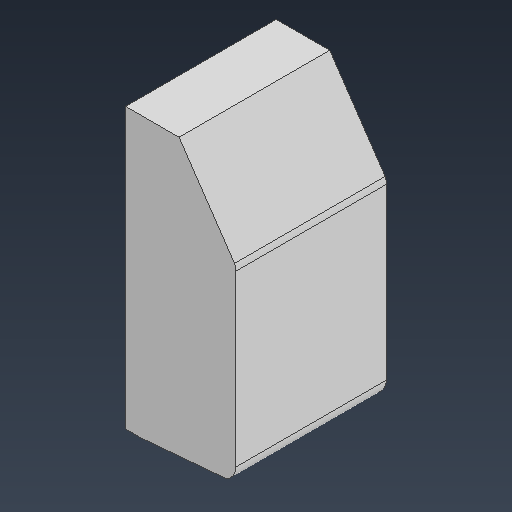
# Autodesk Inventor part: говно деда
Saved by Autodesk Inventor 2025 (Build 290162000, 162)
## iProperties
Created: 2025-03-14
Part Number: говно деда
Material: Типовые
Document SubType Name: Modeling
Designer: GameHD
Density: 1 g/cm^3
Appearance: По умолчанию
Author: GameHD
Autodesk Inventor part; units mm, degrees
ref_plane "YZ Plane" through (0, 0, 0) normal (1, 0, 0) x (0, 1, 0)
ref_plane "XZ Plane" through (0, 0, 0) normal (0, 1, 0) x (-1, 0, 0)
ref_plane "XY Plane" through (0, 0, 0) normal (0, 0, 1) x (1, 0, 0)
sketch "Эскиз1" plane through (0, 0, 0) normal (0, 0, 1) x (1, 0, 0)
  line L0 (-34.5939, -55.1342) -> (-34.5939, -82.0742)
  line L1 (-34.5939, -82.0742) -> (-25.3439, -82.0742)
  line L2 (-25.3439, -82.0742) -> (27.5337, -77.5454)
  arc A0 (27.5337, -77.5454) -> (33.4061, -68.437) centre (23.4061, -68.437) ccw
  line L3 (33.4061, -68.437) -> (33.4061, 36.4028)
  arc A1 (33.4061, 36.2488) -> (30.4771, 43.3199) centre (23.4061, 36.2488) ccw
  line L4 (-16.5939, 90.3909) -> (-34.5939, 90.3909)
  line L5 (-34.5939, 90.3909) -> (-34.5939, 72.3909)
  line L6 (-26.5939, 80.3909) -> (-26.3439, 80.3909)
  line L7 (-34.5939, 90.3909) -> (-34.5939, -82.0742)
  line L8 (-16.5939, 90.3909) -> (-1.5875, 90.3909)
  line L9 (-1.5875, 90.3909) -> (32.6449, 40.0756)
  line L10 (-1.5875, 80.3909) -> (-29.9689, 80.3909)
  line L11 (-29.9689, 80.3909) -> (-29.9689, -77.5454)
  line L12 (-29.9689, -77.5454) -> (19.05, -73.3471)
  line L13 (19.05, -73.3471) -> (23.4061, -68.437)
  line L14 (23.4061, -68.437) -> (23.4061, 36.2488)
  line L15 (23.4061, 36.2488) -> (-1.5875, 80.3909)
  point P0 (0, 0)
  point P1 (22.0964, -89.1509)
  point P2 (33.4061, 36.2488)
  constraints: 32 end point, 5 point on circle, 3 parallel, 2 centre point, 2 horizontal, 1 collinear
extrude "Выдавливание1" add sketch "Эскиз1" along normal blind 90
sketch "Эскиз2" plane through (0, 0, 90) normal (0, 0, 1) x (1, 0, 0)
  line L0 (-1.5875, 90.3909) -> (-34.5939, 90.3909) projected
  line L1 (-34.5939, 90.3909) -> (-34.5939, -82.0742) projected
  line L2 (-34.5939, -82.0742) -> (-25.3439, -82.0742) projected
  line L3 (-25.3439, -82.0742) -> (27.5337, -77.5454) projected
  arc A0 (27.5337, -77.5454) -> (33.4061, -68.437) centre (23.4061, -68.437) ccw projected
  line L4 (33.4061, -68.437) -> (33.4061, 36.2488) projected
  arc A1 (33.4061, 36.2488) -> (32.6449, 40.0756) centre (23.4061, 36.2488) ccw projected
  line L5 (32.6449, 40.0756) -> (-1.5875, 90.3909) projected
  line L6 (-1.5875, 80.3909) -> (23.4061, 36.2488) projected
  line L7 (23.4061, 36.2488) -> (23.4061, -68.437) projected
  line L8 (23.4061, -68.437) -> (19.05, -73.3471) projected
  line L9 (19.05, -73.3471) -> (-29.9689, -77.5454) projected
  line L10 (-29.9689, -77.5454) -> (-29.9689, 80.3909) projected
  line L11 (-29.9689, 80.3909) -> (-1.5875, 80.3909) projected
  point P0 (0, 0)
extrude "Выдавливание2" add sketch "Эскиз2" along normal blind 3 contours L5 A1 L4 A0 L3 L2 L1 L0 | L6 L7 L8 L9 L10 L11
